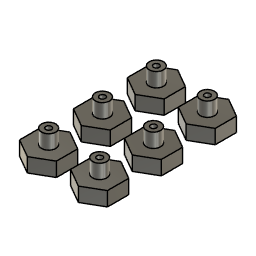
Wheel-Connectors (Autodesk Fusion 360 design; units mm, degrees)
Autodesk Fusion 360 part; units mm, degrees
sketch "Sketch1" plane through (0, 0, 0) normal (0, 0, 1) x (1, 0, 0)
  circle A0 centre (0, 0) radius 7.5
  line L0 (0, 7.5) -> (-6.4952, 3.75)
  line L1 (-6.4952, 3.75) -> (-6.4952, -3.75)
  line L2 (-6.4952, -3.75) -> (0, -7.5)
  line L3 (0, -7.5) -> (6.4952, -3.75)
  line L4 (6.4952, -3.75) -> (6.4952, 3.75)
  line L5 (6.4952, 3.75) -> (0, 7.5)
  circle A1 centre (0, 0) radius 2.5
  circle A2 centre (0, 0) radius 1
  dimension "d1" = 15
  dimension "d2" = 5
  dimension "d3" = 2
  constraint coincident A0.centre A1.centre
  constraint coincident A0 L0.start
  constraint concentric A0 A2
  measures "d1" diameter of A0
  measures "d2" diameter of A1
  measures "d3" diameter of A2
extrude "Extrude1" add sketch "Sketch1" along normal blind 5 contours L0 L1 L2 L3 L4 L5 | A1 makes body 1
extrude "Extrude2" add sketch "Sketch1" along normal blind 5 from surface at 5 contours A1 bodies 1
move_body "Move1" bodies 1 to x (1, 0, 0) y (0, 1, 0) z (0, 0, 1) at (10.4209, 10.8636, 0)
copy_body "CopyPasteBodies1" bodies 1 makes body 2
move_body "Move2" bodies 2 to x (1, 0, 0) y (0, 1, 0) z (0, 0, 1) at (18, 0, 0)
copy_body "CopyPasteBodies2" bodies 1 2 makes body 3 makes body 4
move_body "Move3" bodies 3 4 to x (1, 0, 0) y (0, 1, 0) z (0, 0, 1) at (0, 19, 0)
copy_body "CopyPasteBodies3" bodies 4 3 makes body 5 makes body 6
move_body "Move4" bodies 5 6 to x (1, 0, 0) y (0, 1, 0) z (0, 0, 1) at (0, 20, 0)
move_body "Move5" bodies 6 5 to x (1, 0, 0) y (0, 1, 0) z (0, 0, 1) at (0, -1, 0)
